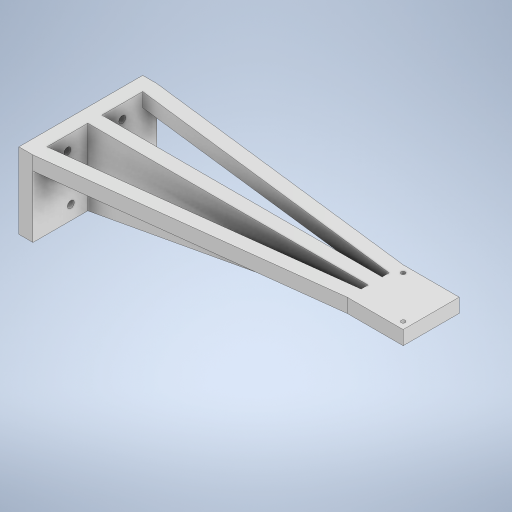
# Autodesk Inventor part: magnetometer_holder
Saved by Autodesk Inventor 2024 (Build 280153000, 153)
## iProperties
Created: 2026-01-01
Part Number: magnetometer_holder
Material: PET Plastic
Document SubType Name: Modeling
Designer: schar
Density: 1.541 g/cm^3
Appearance: Polycarbonate - Clear
Author: schar
Autodesk Inventor part; units mm, degrees
ref_plane "YZ Plane" through (0, 0, 0) normal (1, 0, 0) x (0, 1, 0)
ref_plane "XZ Plane" through (0, 0, 0) normal (0, 1, 0) x (-1, 0, 0)
sketch "Sketch1" plane through (0, 0, 0) normal (0, 1, 0) x (-1, 0, 0)
  line L0 (20, 20) -> (-20, 20)
  line L1 (-20, 20) -> (-20, -20)
  line L2 (-20, -20) -> (20, -20)
  line L3 (20, -20) -> (20, 20)
  line L4 (20, 20) -> (-20, -20) construction
  line L5 (-20, 20) -> (20, -20) construction
  line L6 (-20, 0) -> (230, 0)
  line L7 (230, 0) -> (230, 44.15)
  line L8 (230, 44.15) -> (220, 44.15)
  line L9 (220, 44.15) -> (230, 44.15)
  line L10 (230, 44.15) -> (230, -44.15)
  line L11 (230, -44.15) -> (220, -44.15)
  line L12 (220, -44.15) -> (220, 44.15)
  line L13 (220, 44.15) -> (20, 20)
  line L14 (220, -44.15) -> (20, -20)
  line L15 (20, -20) -> (20, -10)
  line L16 (20, 20) -> (20, 10)
  line L17 (220, 44.15) -> (220, 34.15)
  line L18 (220, -44.15) -> (220, -34.15)
  line L19 (20, 10) -> (220, 34.15)
  line L20 (220, -34.15) -> (20, -10)
  line L21 (220, 0) -> (220, -5)
  line L22 (20, 0) -> (20, 5)
  line L23 (220, -5) -> (20, -5)
  line L24 (20, -5) -> (20, 5)
  line L25 (20, 5) -> (220, 5)
  line L26 (220, 5) -> (220, -5)
  line L27 (-20, 20) -> (-20, 15)
  line L28 (-20, 15) -> (-15, 15)
  line L29 (20, -20) -> (15, -20)
  line L30 (15, -20) -> (15, -15)
  circle A0 centre (15, -15) radius 1.5
  circle A1 centre (-15, 15) radius 1.5
  point P0 (0, 0)
  dimension "d0" = 40
  dimension "d1" = 40
  dimension "d2" = 250
  dimension "d3" = 44.15
  dimension "d4" = 10
  dimension "d5" = 88.3
  dimension "d6" = 10
  dimension "d7" = 10
  dimension "d8" = 10
  dimension "d9" = 10
  dimension "d10" = 5
  dimension "d11" = 5
  dimension "d12" = 5
  dimension "d13" = 5
  dimension "d14" = 3
  dimension "d15" = 3
  constraints: 62 end point, 10 point on line, 6 parallel, 5 horizontal, 5 midpoint, 5 perpendicular, 2 centre point, 2 coincident, 1 vertical
  measures "d0" distance of L2.end L1.end
  measures "d1" distance of L1.end L0.end
  measures "d2" distance of L6.start L6.end
  measures "d3" distance of L6.end L7.end
  measures "d4" distance of L7.end L8.end
  measures "d5" distance of L9.end L10.end
  measures "d6" distance of L2.end L15.end
  measures "d7" distance of L0.start L16.end
  measures "d8" distance of L8.end L17.end
  measures "d9" distance of L11.end L18.end
  measures "d10" distance of L21.start L21.end
  measures "d11" distance of L22.start L22.end
  measures "d12" distance of L0.end L27.end
  measures "d13" distance of L2.end L29.end
  measures "d14" diameter of A0
  measures "d15" diameter of A1
extrude "Extrusion1" add sketch "Sketch1" against normal blind 10 contours L3 L6 L1 L0 | L13 L12 L19 L3 | L8 L7 L6 L12 | L25 L12 L6 L3 | L6 L3 L2 L1 | L6 L12 L23 L3 | L10 L11 L12 L6 | L20 L12 L14 L3
sketch "Sketch2" plane through (0, -10, 0) normal (0, -1, 0) x (1, 0, 0)
  line L0 (-230, 44.15) -> (-230, -44.15) projected
  line L1 (-230, 44.15) -> (-220, 44.15) projected
  line L2 (-230, -44.15) -> (-220, -44.15)
  line L3 (-220, -44.15) -> (-220, 44.15)
  line L4 (-220, 44.15) -> (-230, 44.15)
  line L5 (-230, 44.15) -> (-230, -44.15)
  point P0 (0, 0)
  constraints: 8 end point, 2 parallel, 1 horizontal, 1 perpendicular
extrude "Extrusion2" add sketch "Sketch2" along normal blind 44.112
ref_plane "Work Plane1" through (-220, 0, 5) normal (0, 0, 1) x (1, 0, 0)
sketch "Sketch3" plane through (-220, 0, 5) normal (0, 0, 1) x (1, 0, 0)
  line L0 (0, -10) -> (0, -54.112) projected
  line L1 (200, -10) -> (240, -10) projected
  line L2 (0, -54.112) -> (240, -10)
  line L3 (0, 0) -> (0, -10) projected
  line L4 (0, -54.112) -> (0, -10)
  line L5 (0, -10) -> (240, -10)
  point P0 (220, 0)
  constraints: 6 end point, 1 perpendicular, 1 vertical
extrude "Extrusion3" add sketch "Sketch3" against normal blind 10
sketch "Sketch5" plane through (-220, 0, 34.15) normal (1, 0, 0) x (0, 0, -1)
  line L0 (0, 0) -> (29.15, 0) projected
  line L1 (0, 0) -> (14.575, 0)
  line L2 (14.575, 0) -> (14.575, -10)
  circle A0 centre (14.575, -10) radius 2.5
  line L3 (34.15, 0) -> (34.15, -54.112)
  line L4 (39.15, -54.112) -> (29.15, -54.112) projected
  circle A1 centre (53.725, -10) radius 2.5
  dimension "d23" = 14.575
  dimension "d24" = 10
  dimension "d25" = 5
  constraints: 6 end point, 2 centre point, 2 midpoint, 1 coincident, 1 perpendicular, 1 symmetric about line, 1 other
  measures "d23" distance of L0.start L1.end
  measures "d24" distance of L1.end L2.end
  measures "d25" diameter of A0
extrude "Extrusion4" cut sketch "Sketch5" against normal blind 10
sketch "Sketch6" plane through (-220, 0, 34.15) normal (1, 0, 0) x (0, 0, -1)
  line L0 (-10, 0) -> (-10, -54.112) projected
  line L1 (-10, -54.112) -> (17, -54.112)
  line L2 (17, -54.112) -> (17, -44.112)
  circle A0 centre (17, -44.112) radius 2.5
  line L3 (34.15, 0) -> (34.15, -54.112)
  line L4 (39.15, -54.112) -> (29.15, -54.112) projected
  circle A1 centre (51.3, -44.112) radius 2.5
  dimension "d28" = 27
  dimension "d29" = 10
  dimension "d30" = 5
  constraints: 6 end point, 2 centre point, 1 coincident, 1 horizontal, 1 midpoint, 1 perpendicular, 1 symmetric about line, 1 other
  measures "d28" distance of L0.end L1.end
  measures "d29" distance of L1.end L2.end
  measures "d30" diameter of A0
extrude "Extrusion5" cut sketch "Sketch6" against normal blind 10
body "Solid1"
